Screen 4-3 (Autodesk Fusion 360 design; units mm, degrees)
part number: Screen 4-3
Autodesk Fusion 360 part; units mm, degrees
sketch "Sketch1" plane through (0, 0, 0) normal (0, 0, 1) x (1, 0, 0)
  line L0 (18, 0) -> (170, 0)
  line L1 (188, 18) -> (188, 151)
  line L2 (188, 151) -> (0, 151)
  line L3 (0, 151) -> (0, 18)
  arc A0 (170, 0) -> (188, 18) centre (170, 18) ccw
  arc A1 (0, 18) -> (18, 0) centre (18, 18) ccw
  line L4 (186, 20) -> (186, 148)
  line L5 (186, 148) -> (2, 148)
  line L6 (2, 148) -> (2, 20)
  arc A2 (2, 20) -> (18, 4) centre (18, 20) ccw
  line L7 (18, 4) -> (170, 4)
  arc A3 (170, 4) -> (186, 20) centre (170, 20) ccw
  line L8 (16, 138) -> (171, 138)
  line L9 (176, 133) -> (176, 19)
  line L10 (171, 14) -> (16, 14)
  line L11 (11, 19) -> (11, 133)
  arc A4 (176, 133) -> (171, 138) centre (171, 133) ccw
  arc A5 (16, 138) -> (11, 133) centre (16, 133) ccw
  arc A6 (11, 19) -> (16, 14) centre (16, 19) ccw
  arc A7 (171, 14) -> (176, 19) centre (171, 19) ccw
  arc A8 (182, 133) -> (171, 144) centre (171, 133) ccw
  line L12 (16, 144) -> (171, 144)
  arc A9 (16, 144) -> (5, 133) centre (16, 133) ccw
  line L13 (5, 19) -> (5, 133)
  arc A10 (5, 19) -> (16, 8) centre (16, 19) ccw
  line L14 (171, 8) -> (16, 8)
  arc A11 (171, 8) -> (182, 19) centre (171, 19) ccw
  line L15 (182, 133) -> (182, 19)
  line L16 (300.3936, 142.6585) -> (455.3936, 142.6585)
  arc A12 (466.3936, 131.6585) -> (455.3936, 142.6585) centre (455.3936, 131.6585) ccw
  line L17 (466.3936, 131.6585) -> (466.3936, 17.6585)
  arc A13 (455.3936, 6.6585) -> (466.3936, 17.6585) centre (455.3936, 17.6585) ccw
  line L18 (455.3936, 6.6585) -> (300.3936, 6.6585)
  arc A14 (289.3936, 17.6585) -> (300.3936, 6.6585) centre (300.3936, 17.6585) ccw
  line L19 (289.3936, 17.6585) -> (289.3936, 131.6585)
  arc A15 (300.3936, 142.6585) -> (289.3936, 131.6585) centre (300.3936, 131.6585) ccw
  arc A16 (470.3936, 131.6585) -> (455.3936, 146.6585) centre (455.3936, 131.6585) ccw
  line L20 (300.3936, 146.6585) -> (455.3936, 146.6585)
  arc A17 (300.3936, 146.6585) -> (285.3936, 131.6585) centre (300.3936, 131.6585) ccw
  line L21 (285.3936, 17.6585) -> (285.3936, 131.6585)
  arc A18 (285.3936, 17.6585) -> (300.3936, 2.6585) centre (300.3936, 17.6585) ccw
  line L22 (455.3936, 2.6585) -> (300.3936, 2.6585)
  arc A19 (455.3936, 2.6585) -> (470.3936, 17.6585) centre (455.3936, 17.6585) ccw
  line L23 (470.3936, 131.6585) -> (470.3936, 17.6585)
  point P0 (188, 0)
  point P1 (11, 138)
  point P2 (176, 138)
  point P3 (11, 14)
  dimension "d1" = 188
  dimension "d2" = 151
  dimension "d3" = 18
  dimension "d55" = 165
  dimension "d56" = 124
  dimension "d57" = 13
  dimension "d58" = 12
  dimension "d59" = 5
  dimension "d60" = -6
  dimension "d82" = -4
  constraint horizontal L0
  constraint vertical L1
  constraint horizontal L2
  constraint vertical L3
  constraint coincident P0 L0
  constraint coincident P0 L1
  constraint tangent L0 A0
  constraint tangent L1 A0
  constraint coincident origin L0
  constraint coincident origin L3
  constraint tangent L0 A1
  constraint tangent L3 A1
  constraint equal A0 A1
  constraint parallel L1 L4
  constraint parallel L2 L5
  constraint parallel L3 L6
  constraint horizontal L8
  constraint vertical L9
  constraint horizontal L10
  constraint vertical L11
  constraint coincident P2 L8
  constraint coincident P2 L9
  constraint tangent L8 A4
  constraint tangent L9 A4
  constraint coincident P1 L8
  constraint coincident P1 L11
  constraint tangent L8 A5
  constraint tangent L11 A5
  constraint equal A4 A5
  constraint coincident P3 L10
  constraint coincident P3 L11
  constraint tangent L10 A6
  constraint tangent L11 A6
  constraint equal A4 A6
  constraint tangent L9 A7
  constraint tangent L10 A7
  constraint equal A4 A7
  measures "d1" distance of origin P0
  measures "d2" distance of origin L2.end
  measures "d3" radius of A0
  measures "d55" distance of P1 P2
  measures "d56" distance of P1 P3
  measures "d57" distance of L2 L8
  measures "d58" distance of L1 L9
  measures "d59" radius of A4
extrude "Extrude13" add sketch "Sketch1" along normal blind 3 contours A16 L20 A17 L21 A18 L22 A19 L23 makes body 1
extrude "Extrude8" add sketch "Sketch1" along normal blind 2 separate body contours L0 L1 L2 L3 A0 A1 makes body 2
extrude "Extrude9" add sketch "Sketch1" along normal blind 10 contours L4 L5 L6 A2 L7 A3 | L8 L9 L10 L11 A4 A5 A6 A7 | A8 L12 A9 L13 A10 L14 A11 L15 bodies 2
extrude "Extrude10" cut sketch "Sketch1" along normal blind 10 draft -32 contours L8 L9 L10 L11 A4 A5 A6 A7 | A8 L12 A9 L13 A10 L14 A11 L15 bodies 2
sketch "Sketch7" plane through (0, 0, 10) normal (0, 0, 1) x (-1, 0, 0)
  line L0 (-16, -137.7513) -> (-171, -137.7513)
  arc A0 (-175.7513, -133) -> (-171, -137.7513) centre (-171, -133) ccw
  line L1 (-175.7513, -133) -> (-175.7513, -19)
  arc A1 (-171, -14.2487) -> (-175.7513, -19) centre (-171, -19) ccw
  line L2 (-171, -14.2487) -> (-16, -14.2487)
  arc A2 (-11.2487, -19) -> (-16, -14.2487) centre (-16, -19) ccw
  line L3 (-11.2487, -19) -> (-11.2487, -133)
  arc A3 (-16, -137.7513) -> (-11.2487, -133) centre (-16, -133) ccw
  arc A4 (-170, -4) -> (-186, -20) centre (-170, -20) ccw
  line L4 (-186, -20) -> (-186, -148)
  line L5 (-186, -148) -> (-2, -148)
  line L6 (-2, -148) -> (-2, -20)
  arc A5 (-2, -20) -> (-18, -4) centre (-18, -20) ccw
  line L7 (-18, -4) -> (-170, -4)
  line L8 (-8.3, -146.95) -> (-182.5, -146.95)
  line L9 (-182.5, -146.95) -> (-182.5, -10.75)
  line L10 (-182.5, -10.75) -> (-8.3, -10.75)
  line L11 (-8.3, -10.75) -> (-8.3, -146.95)
  line L12 (-176, -133) -> (-176, -19)
  line L13 (-171, -14) -> (-16, -14)
  dimension "d67" = 174.2
  dimension "d68" = 136.2
  dimension "d69" = 6.5
  dimension "d70" = 3.25
  constraint horizontal L8
  constraint vertical L9
  constraint horizontal L10
  constraint vertical L11
  measures "d67" distance of L8.start L8.end
  measures "d68" distance of L8.start L10.end
  measures "d69" distance of L9 L12
  measures "d70" distance of L10 L13
extrude "Extrude11" add sketch "Sketch7" along normal blind 3 contours A4 L4 L5 L6 A5 L7 bodies 2
move_face "OffsetFaces1" offset 4 1 faces at (63.3333, 148, 9.3333) on bodies 2
fillet "Fillet3" radius 1 1 edges at (94, 152, 2) on bodies 2
fillet "Fillet4" radius 2 8 edges at (470.3936, 74.6585, 3) (466.0002, 142.2651, 3) (377.8936, 146.6585, 3) (289.787, 142.2651, 3) (285.3936, 74.6585, 3) (289.787, 7.0519, 3) (377.8936, 2.6585, 3) (466.0002, 7.0519, 3) on bodies 1
fillet "Fillet5" radius 2 8 edges at (377.8936, 142.6585, 3) (463.1718, 139.4367, 3) (466.3936, 74.6585, 3) (463.1718, 9.8803, 3) (377.8936, 6.6585, 3) (292.6154, 9.8803, 3) (289.3936, 74.6585, 3) (292.6154, 139.4367, 3) on bodies 1
